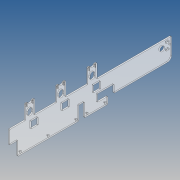
# Autodesk Inventor part: 103.017.01_Wand_Foerderband
Saved by Autodesk Inventor 2021 (Build 250183000, 183)
## iProperties
Created: 2021-11-29
Part Number: 103.017.01_Wand_Foerderband
Material: PMMA-Kunststoff
Document SubType Name: Modeling
Designer: Oliver Ungerer
Density: 1.188 g/cm^3
Appearance: Wasserblasen
Mass: 336.148 g
Surface Area: 1278.3 cm^2
Volume: 282.953 cm^3
Author: Oliver Ungerer
Autodesk Inventor part; units mm, degrees
ref_plane "YZ Plane" through (0, 0, 0) normal (1, 0, 0) x (0, 1, 0)
ref_plane "XZ Plane" through (0, 0, 0) normal (0, 1, 0) x (-1, 0, 0)
ref_plane "XY Plane" through (0, 0, 0) normal (0, 0, 1) x (1, 0, 0)
sketch "Skizze1" plane through (0, 0, 0) normal (1, 0, 0) x (0, 1, 0)
  line L0 (105, 0) -> (53, 0)
  line L1 (53, 0) -> (53, -34)
  line L2 (53, -34) -> (0, -34)
  line L3 (0, -34) -> (0, -268)
  line L4 (0, -268) -> (53, -268)
  line L5 (53, -268) -> (53, -290)
  line L6 (53, -290) -> (0, -290)
  line L7 (25, -380) -> (25, -625.3)
  line L8 (25, -625.3) -> (105, -625.3)
  line L9 (0, -290) -> (0, -380)
  line L10 (0, -380) -> (25, -380)
  line L11 (160, -63.4) -> (105, -63.4)
  line L12 (105, -98.4) -> (160, -98.4)
  line L13 (160, -98.4) -> (160, -63.4)
  line L14 (105, 0) -> (105, -63.4)
  line L15 (160, -183.4) -> (105, -183.4)
  line L16 (105, -218.4) -> (160, -218.4)
  line L17 (160, -218.4) -> (160, -183.4)
  line L18 (160, -303.4) -> (105, -303.4)
  line L19 (105, -338.4) -> (160, -338.4)
  line L20 (160, -338.4) -> (160, -303.4)
  line L21 (105, -98.4) -> (105, -183.4)
  line L22 (105, -218.4) -> (105, -303.4)
  line L23 (105, -338.4) -> (105, -625.3)
  point P0 (0, 0)
  dimension "d0" = 53
  dimension "d1" = 34
  dimension "d2" = 52
  dimension "d3" = 234
  dimension "d4" = 22
  dimension "d6" = 335.3
  dimension "d21" = 90
  dimension "d22" = 25
  dimension "d34" = 35
  dimension "d35" = 63.4
  dimension "d36" = 55
  dimension "d53" = 120
  constraints: 48 end point, 7 vertical, 6 point on line, 5 horizontal, 4 perpendicular, 1 collinear, 1 parallel, 14 other
  measures "d0" distance of L1.end L2.end
  measures "d1" distance of L0.end L1.end
  measures "d2" distance of L0.start L0.end
  measures "d3" distance of L2.end L3.end
  measures "d4" distance of L4.end L5.end
  measures "d6" distance between parallel lines of L6 L8
  measures "d21" distance of L9.start L9.end
  measures "d22" distance between parallel lines of L3 L7
  measures "d34" distance between parallel lines of L11 L12
  measures "d35" distance between parallel lines of L0 L11
  measures "d36" distance between parallel lines of L14 L13
  measures "d53" distance of L11.end L15.end
extrude "Extrusion1" add sketch "Skizze1" along normal blind 5
fillet "Rundung1" radius 15 1 edges at (2.5, 25, -625.3)
sketch "Skizze2" plane through (5, 0, 0) normal (1, 0, 0) x (0, 0, -1)
  line L0 (34, 0) -> (268, 0) projected
  line L1 (34, 53) -> (34, 0) projected
  line L2 (290, 53) -> (290, 0) projected
  line L3 (380, 0) -> (380, 25) projected
  line L4 (268, 0) -> (268, 53) projected
  point P0 (0, 0)
  point P1 (44, 10)
  point P2 (151, 10)
  point P3 (258, 10)
  point P4 (300, 10)
  point P5 (370, 10)
  point P6 (300, 10)
  point P7 (370, 10)
  dimension "d10" = 10
  dimension "d11" = 10
  dimension "d12" = 107
  dimension "d13" = 107
  dimension "d58" = 10
  dimension "d59" = 10
  dimension "d204" = 10
  constraints: 4 horizontal alignment, 2 coincident
  measures "d10" distance from line of L0 point (44, 10)
  measures "d11" distance from line of L1 point (44, 10)
  measures "d12" distance of point (151, 10) point (44, 10)
  measures "d13" distance of point (151, 10) point (258, 10)
  measures "d58" distance from line of L2 point (300, 10)
  measures "d59" distance from line of point (370, 10) L3
  measures "d204" distance from line of L4 point (258, 10)
hole "Bohrung1" at (5, 10, -44) at (5, 10, -151) at (5, 10, -258) at (5, 10, -300) at (5, 10, -370) direction (-1, 0, 0) diameter 4.5 end through all countersink diameter 8.6 countersink angle 90
sketch "Skizze5" plane through (5, 0, 0) normal (1, 0, 0) x (0, 0, -1)
  line L0 (340, 55) -> (404, 55)
  line L1 (380, 27) -> (340, 27)
  line L2 (340, 27) -> (340, 55)
  line L3 (290, 53) -> (290, 0) projected
  line L4 (380, 25) -> (610.3, 25) projected
  line L5 (380, 0) -> (380, 25) projected
  line L6 (380, 25) -> (380, 27)
  line L7 (404, 55) -> (404, 25)
  line L8 (380, 25) -> (404, 25)
  point P0 (0, 0)
  dimension "d65" = 2
  dimension "d172" = 30
  dimension "d173" = 24
  dimension "d174" = 64
  constraints: 12 end point, 2 collinear, 1 horizontal, 1 parallel, 1 perpendicular, 1 point on line
  measures "d65" distance between parallel lines of L4 L1
  measures "d172" distance between parallel lines of L4 L0
  measures "d173" distance between parallel lines of L6 L7
  measures "d174" distance between parallel lines of L7 L2
extrude "Extrusion2" cut sketch "Skizze5" against normal through all
sketch "Skizze6" plane through (5, 0, 0) normal (1, 0, 0) x (0, 0, -1)
  line L0 (84.15, 91.75) -> (111.15, 91.75)
  line L1 (111.15, 91.75) -> (111.15, 66.25)
  line L2 (111.15, 66.25) -> (84.15, 66.25)
  line L3 (84.15, 66.25) -> (84.15, 91.75)
  line L4 (84.15, 91.75) -> (111.15, 66.25) construction
  line L5 (111.15, 91.75) -> (84.15, 66.25) construction
  line L6 (183.4, 105) -> (98.4, 105) projected
  line L7 (98.4, 105) -> (98.4, 160) projected
  line L8 (204.15, 91.75) -> (231.15, 91.75)
  line L9 (231.15, 91.75) -> (231.15, 66.25)
  line L10 (231.15, 66.25) -> (204.15, 66.25)
  line L11 (204.15, 66.25) -> (204.15, 91.75)
  line L12 (204.15, 91.75) -> (231.15, 66.25) construction
  line L13 (231.15, 91.75) -> (204.15, 66.25) construction
  line L14 (324.15, 91.75) -> (351.15, 91.75)
  line L15 (351.15, 91.75) -> (351.15, 66.25)
  line L16 (351.15, 66.25) -> (324.15, 66.25)
  line L17 (324.15, 66.25) -> (324.15, 91.75)
  line L18 (324.15, 91.75) -> (351.15, 66.25) construction
  line L19 (351.15, 91.75) -> (324.15, 66.25) construction
  point P0 (0, 0)
  point P1 (97.65, 79)
  point P2 (217.65, 79)
  point P3 (337.65, 79)
  dimension "d68" = 27
  dimension "d69" = 25.5
  dimension "d70" = 26
  dimension "d79" = 120
  dimension "d202" = 0.75
  constraints: 36 end point, 6 midpoint, 2 horizontal, 2 parallel, 1 collinear, 1 perpendicular, 21 other
  measures "d68" distance of L0.start L0.end
  measures "d69" distance between parallel lines of L2 L0
  measures "d70" distance from line of point (97.65, 79) L6
  measures "d79" distance of L0.start L8.start
  measures "d202" distance from line of L7 point (97.65, 79)
extrude "Extrusion3" cut sketch "Skizze6" against normal blind 5
sketch "Skizze7" plane through (5, 0, 0) normal (1, 0, 0) x (0, 0, -1)
  arc A0 (90.05, 129) -> (71.75, 129) centre (80.9, 129) ccw
  line L0 (63.4, 160) -> (63.4, 105) projected
  line L1 (63.4, 105) -> (0, 105) projected
  arc A1 (71.75, 121) -> (90.05, 121) centre (80.9, 121) ccw
  line L2 (90.05, 129) -> (90.05, 121)
  line L3 (71.75, 129) -> (71.75, 121)
  arc A2 (210.05, 129) -> (191.75, 129) centre (200.9, 129) ccw
  arc A3 (191.75, 121) -> (210.05, 121) centre (200.9, 121) ccw
  line L4 (210.05, 129) -> (210.05, 121)
  line L5 (191.75, 129) -> (191.75, 121)
  arc A4 (330.05, 129) -> (311.75, 129) centre (320.9, 129) ccw
  arc A5 (311.75, 121) -> (330.05, 121) centre (320.9, 121) ccw
  line L6 (330.05, 129) -> (330.05, 121)
  line L7 (311.75, 129) -> (311.75, 121)
  point P0 (0, 0)
  dimension "d85" = 17.5
  dimension "d89" = 24
  dimension "d132" = 18.3
  dimension "d133" = 8
  dimension "d143" = 120
  constraints: 12 end point, 12 point on circle, 6 centre point, 4 tangent, 1 equal radius, 1 horizontal, 1 vertical, 20 other
  measures "d85" distance from line of A0.centre L0
  measures "d89" distance from line of A0.centre L1
  measures "d132" diameter of A1
  measures "d133" distance of A1.centre A0.centre
  measures "d143" distance of A0.centre A2.centre
extrude "Extrusion4" cut sketch "Skizze7" against normal through all
fillet "Rundung2" radius 2 15 edges at (2.5, 53, -34) (2.5, 53, -268) (2.5, 53, -290) (2.5, 55, -340) (2.5, 27, -340) (2.5, 55, -404) (2.5, 53, 0) (2.5, 105, 0) (2.5, 0, -34) (2.5, 0, -268) (2.5, 0, -290) (2.5, 0, -380) (2.5, 105, -625.3) (2.5, 27, -380) (2.5, 25, -404)
fillet "Rundung2" radius 2 12 edges at (2.5, 105, -338.4) (2.5, 160, -338.4) (2.5, 160, -303.4) (2.5, 105, -303.4) (2.5, 105, -218.4) (2.5, 160, -218.4) (2.5, 160, -183.4) (2.5, 105, -183.4) (2.5, 105, -98.4) (2.5, 160, -98.4) (2.5, 160, -63.4) (2.5, 105, -63.4)
sketch "Skizze9" plane through (0, 0, 0) normal (-1, 0, 0) x (0, 0, 1)
  arc A0 (-90.65, 156) -> (-94.15, 156) centre (-92.4, 156) ccw
  arc A1 (-71.75, 129) -> (-90.05, 129) centre (-80.9, 129) ccw projected
  arc A2 (-94.15, 148) -> (-90.65, 148) centre (-92.4, 148) ccw
  line L0 (-94.15, 148) -> (-94.15, 156)
  line L1 (-90.65, 148) -> (-90.65, 156)
  line L2 (-80.9, 129) -> (-80.9, 159.9245)
  arc A3 (-67.65, 156) -> (-71.15, 156) centre (-69.4, 156) ccw
  arc A4 (-71.15, 148) -> (-67.65, 148) centre (-69.4, 148) ccw
  line L3 (-67.65, 148) -> (-67.65, 156)
  line L4 (-71.15, 148) -> (-71.15, 156)
  line L5 (-96.4, 160) -> (-65.4, 160) projected
  arc A5 (-191.15, 148) -> (-187.65, 148) centre (-189.4, 148) ccw
  line L6 (-187.65, 148) -> (-187.65, 156)
  line L7 (-191.15, 148) -> (-191.15, 156)
  line L8 (-214.15, 148) -> (-214.15, 156)
  arc A6 (-214.15, 148) -> (-210.65, 148) centre (-212.4, 148) ccw
  arc A7 (-187.65, 156) -> (-191.15, 156) centre (-189.4, 156) ccw
  arc A8 (-210.65, 156) -> (-214.15, 156) centre (-212.4, 156) ccw
  line L9 (-210.65, 148) -> (-210.65, 156)
  arc A9 (-311.15, 148) -> (-307.65, 148) centre (-309.4, 148) ccw
  line L10 (-307.65, 148) -> (-307.65, 156)
  line L11 (-311.15, 148) -> (-311.15, 156)
  line L12 (-334.15, 148) -> (-334.15, 156)
  arc A10 (-334.15, 148) -> (-330.65, 148) centre (-332.4, 148) ccw
  arc A11 (-307.65, 156) -> (-311.15, 156) centre (-309.4, 156) ccw
  arc A12 (-330.65, 156) -> (-334.15, 156) centre (-332.4, 156) ccw
  line L13 (-330.65, 148) -> (-330.65, 156)
  point P0 (0, 0)
  point P1 (-200.9, 159.9245)
  point P2 (-185.4, 160)
  point P3 (-216.4, 160)
  point P4 (-320.9, 159.9245)
  point P5 (-305.4, 160)
  point P6 (-336.4, 160)
  dimension "d148" = 3.5
  dimension "d149" = 27
  dimension "d150" = 11.5
  dimension "d151" = 8
  dimension "d154" = 120
  constraints: 26 end point, 24 point on circle, 12 centre point, 6 symmetric about line, 3 vertical, 2 tangent, 1 equal radius, 1 horizontal, 48 other
  measures "d148" diameter of A0
  measures "d149" vertical distance of L2.start A0.centre
  measures "d150" horizontal distance of A0.centre L2.start
  measures "d151" distance of A0.centre A2.centre
  measures "d154" distance of L1.start L9.start
extrude "Extrusion5" cut sketch "Skizze9" against normal through all
sketch "Skizze10" plane through (0, 0, 0) normal (-1, 0, 0) x (0, 0, 1)
  arc A0 (-71.75, 129) -> (-90.05, 129) centre (-80.9, 129) ccw projected
  line L0 (-80.9, 129) -> (-80.9, 163)
  line L1 (-96.4, 160) -> (-65.4, 160) projected
  circle A1 centre (-80.9, 163) radius 9.25
  circle A2 centre (-200.9, 163) radius 9.25
  circle A3 centre (-320.9, 163) radius 9.25
  point P0 (0, 0)
  dimension "d161" = 3
  dimension "d162" = 18.5
  dimension "d165" = 120
  constraints: 3 centre point, 2 end point, 1 coincident, 1 horizontal, 1 vertical, 4 other
  measures "d161" distance from line of L0.end L1
  measures "d162" diameter of A1
  measures "d165" distance of A1.centre A2.centre
extrude "Extrusion6" cut sketch "Skizze10" against normal through all
sketch "Skizze11" plane through (0, 0, 0) normal (-1, 0, 0) x (0, 0, 1)
  line L0 (-615.5, 95.2) -> (-605.1, 95.2)
  line L1 (-605.1, 95.2) -> (-605.1, 89.8)
  line L2 (-605.1, 89.8) -> (-615.5, 89.8)
  line L3 (-615.5, 89.8) -> (-615.5, 95.2)
  line L4 (-625.3, 40) -> (-625.3, 103) projected
  line L5 (-623.3, 105) -> (-340.4, 105) projected
  line L6 (-615.5, 70.2) -> (-605.1, 70.2)
  line L7 (-605.1, 70.2) -> (-605.1, 64.8)
  line L8 (-605.1, 64.8) -> (-615.5, 64.8)
  line L9 (-615.5, 64.8) -> (-615.5, 70.2)
  circle A0 centre (-619.3, 80) radius 2.75
  point P0 (0, 0)
  point P1 (-625.3, 78)
  dimension "d176" = 5.4
  dimension "d177" = 10.4
  dimension "d178" = 9.8
  dimension "d179" = 15.2
  dimension "d182" = 25
  dimension "d187" = 9.8
  dimension "d188" = 6
  dimension "d189" = 5.5
  constraints: 16 end point, 2 parallel, 1 centre point, 1 horizontal, 1 perpendicular, 1 vertical, 9 other
  measures "d176" distance between parallel lines of L2 L0
  measures "d177" distance between parallel lines of L3 L1
  measures "d178" distance between parallel lines of L4 L3
  measures "d179" distance between parallel lines of L5 L2
  measures "d182" distance of L0.start L6.start
  measures "d187" distance from line of A0.centre L2
  measures "d188" distance from line of L4 A0.centre
  measures "d189" diameter of A0
extrude "Extrusion7" cut sketch "Skizze11" against normal through all
fillet "Rundung3" radius 4 6 edges at (2.5, 160, -329.65) (2.5, 160, -312.15) (2.5, 160, -209.65) (2.5, 160, -192.15) (2.5, 160, -89.65) (2.5, 160, -72.15)
sketch "Skizze12" plane through (0, 0, 0) normal (-1, 0, 0) x (0, 0, 1)
  line L0 (-625.3, 40) -> (-625.3, 103) projected
  circle A0 centre (-619.3, 80) radius 2.75 projected
  line L1 (-619.3, 80) -> (-616.55, 80)
  point P0 (0, 0)
  point P1 (-589.7, 80)
  dimension "d193" = 35.6
  constraints: 2 end point, 1 horizontal, 1 horizontal alignment, 1 point on line, 1 other
  measures "d193" distance from line of point (-589.7, 80) L0
hole "Bohrung4" at (0, 80, -589.7) direction (1, 0, 0) diameter 18.5 end through all
fillet "Rundung4" radius 0.5 12 edges at (2.5, 66.25, -84.15) (2.5, 66.25, -111.15) (2.5, 91.75, -111.15) (2.5, 91.75, -84.15) (2.5, 91.75, -204.15) (2.5, 91.75, -231.15) (2.5, 66.25, -231.15) (2.5, 66.25, -204.15) (2.5, 66.25, -351.15) (2.5, 66.25, -324.15) (2.5, 91.75, -324.15) (2.5, 91.75, -351.15)
sketch "Skizze13" plane through (5, 0, 0) normal (1, 0, 0) x (0, 0, -1)
  line L0 (0, 105) -> (2, 105)
  line L1 (2, 105) -> (2, 53)
  line L2 (2, 53) -> (0, 53)
  line L3 (0, 53) -> (0, 105)
  line L4 (61.4, 105) -> (2, 105) projected
  line L5 (2, 53) -> (32, 53) projected
  line L6 (0, 103) -> (0, 55) projected
  point P0 (0, 0)
  dimension "d205" = 2
  constraints: 8 end point, 3 collinear, 2 parallel, 1 horizontal, 1 perpendicular
  measures "d205" distance between parallel lines of L3 L1
extrude "Extrusion8" cut sketch "Skizze13" against normal through all
fillet "Rundung5" radius 2 2 edges at (2.5, 105, -2) (2.5, 53, -2)
